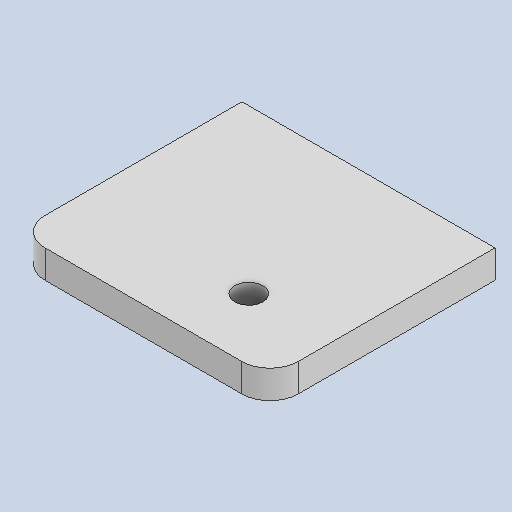
# Autodesk Inventor part: Y-Umlenkrollenhalter
Saved by Autodesk Inventor 2022 (Build 260153000, 153)
## iProperties
Created: 2021-04-27
Part Number: Y-Umlenkrollenhalter
Material: Generic
Document SubType Name: Modeling
Designer: Fabijan_Sven
Density: 1 g/cm^3
Appearance: Default
Author: Fabijan_Sven
Autodesk Inventor part; units mm, degrees
ref_plane "YZ Plane" through (0, 0, 0) normal (1, 0, 0) x (0, 1, 0)
ref_plane "XZ Plane" through (0, 0, 0) normal (0, 1, 0) x (-1, 0, 0)
ref_plane "XY Plane" through (0, 0, 0) normal (0, 0, 1) x (1, 0, 0)
sketch "Sketch1" plane through (0, 0, 0) normal (0, 0, 1) x (1, 0, 0)
  line L0 (-30, -3.3413) -> (15, -3.3413)
  line L1 (15, -3.3413) -> (15, -8.3413)
  line L2 (15, -8.3413) -> (-30, -8.3413)
  line L3 (-30, -8.3413) -> (-30, -3.3413)
  line L4 (-30, -65) -> (-30, 65) projected
  line L5 (15, -7) -> (15, 7) projected
  line L6 (-24.8253, -20.3413) -> (25.1747, -20.3413) projected
  point P0 (0, 0)
  dimension "d0" = 5
  dimension "d1" = 12
  constraints: 8 end point, 2 collinear, 2 parallel, 1 horizontal, 1 perpendicular
  measures "d0" distance of L0.end L1.end
  measures "d1" distance between parallel lines of L2 L6
extrude "Extrusion1" add sketch "Sketch1" along normal blind 40
fillet "Fillet1" radius 5 2 edges at (-30, -5.8413, 40) (15, -5.8413, 40)
sketch "Sketch2" plane through (-30, -3.3413, 0) normal (0, 1, 0) x (1, 0, 0)
  circle A0 centre (30.1747, -28.9529) radius 2.5 projected
  point P0 (30, 0)
hole "Hole1" at (0.1747, -3.3413, 28.9529) direction (0, -1, 0) diameter 5 depth 8 tip angle 118
sketch "Sketch3" plane through (0, 0, 0) normal (0, 0, -1) x (-1, 0, 0)
  circle A0 centre (-10, -6.5) radius 1.5 projected
  circle A1 centre (20, -6.5) radius 1.5 projected
  point P0 (0, 0)
hole "Hole2" at (10, -6.5, 0) at (-20, -6.5, 0) direction (0, 0, 1) diameter 2.459 depth 20 tip angle 118 thread size "M3x0.5" class "6H" standard "ISO Metric profile"
body "Solid1"
